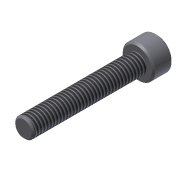
# Autodesk Inventor part: M6 x 12mm
Saved by Autodesk Inventor 2011 SP1 (Build 150282100, 282)
## iProperties
Created: 2011-07-22
Part Number: M6 x 12mm
Material: Steel
Document SubType Name: Modeling
Designer: Dan Niemitalo
Density: 7.85 g/cm^3
Author: Dan Niemitalo
Autodesk Inventor part; units mm, degrees
ref_plane "YZ Plane" through (0, 0, 0) normal (1, 0, 0) x (0, 1, 0)
ref_plane "XZ Plane" through (0, 0, 0) normal (0, 1, 0) x (-1, 0, 0)
ref_plane "XY Plane" through (0, 0, 0) normal (0, 0, 1) x (1, 0, 0)
sketch "Sketch1" plane through (0, 0, 0) normal (0, 0, 1) x (1, 0, 0)
  circle A0 centre (0, 0) radius 3
  dimension "d0" = 6
  constraints: 1 centre point, 1 coincident
  measures "d0" diameter of A0
extrude "Extrusion1" add sketch "Sketch1" along normal blind 35
sketch "Sketch2" plane through (0, 0, 0) normal (0, 0, -1) x (-1, 0, 0)
  circle A0 centre (0, 0) radius 3 projected
  circle A1 centre (0, 0) radius 5
  dimension "d3" = 10
  constraints: 1 centre point, 1 coincident
  measures "d3" diameter of A1
extrude "Extrusion2" add sketch "Sketch2" along normal blind 6 contours A0 | A1
sketch "Sketch3" plane through (0, 0, -6) normal (0, 0, -1) x (-1, 0, 0)
  circle A0 centre (0, 0) radius 5 projected
  line L0 (-1.4434, 2.5) -> (1.4434, 2.5)
  line L1 (1.4434, 2.5) -> (2.8868, 0)
  line L2 (2.8868, 0) -> (1.4434, -2.5)
  line L3 (1.4434, -2.5) -> (-1.4434, -2.5)
  line L4 (-1.4434, -2.5) -> (-2.8868, 0)
  line L5 (-2.8868, 0) -> (-1.4434, 2.5)
  dimension "d6" = 5
  constraints: 12 end point, 1 coincident, 1 horizontal, 13 other
  measures "d6" distance between parallel lines of L3 L0
extrude "Extrusion3" cut sketch "Sketch3" against normal blind 3 contours L0 L1 L2 L3 L4 L5
thread "Thread1" size "M6x1" class "6g" standard "ANSI Metric M Profile" full length
chamfer "Chamfer1" distance 0.508 angle 45 3 edges at (5, 0, -6) (5, 0, 0) (-3, 0, 35)
body "Solid1"
